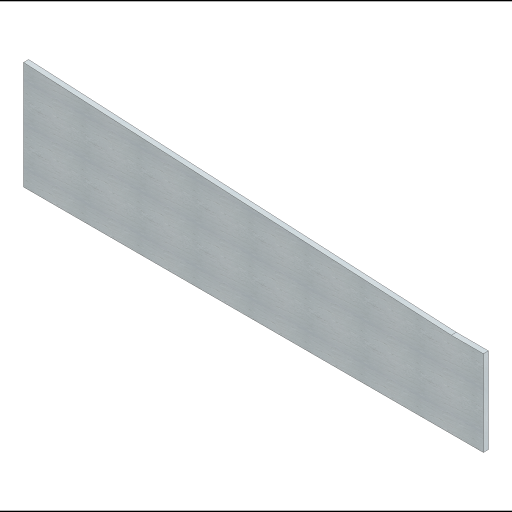
# Autodesk Inventor part: Outlet Support Leg Proto 1
Saved by Autodesk Inventor 2023 (Build 270158000, 158)
## iProperties
Created: 2023-01-19
Part Number: Outlet Support Leg Proto 1
Material: Wood (Oak)
Document SubType Name: Modeling
Designer: kamer
Density: 0.76 g/cm^3
Appearance: Wood - Painted White
Author: kamer
Autodesk Inventor part; units mm, degrees
ref_plane "YZ Plane" through (0, 0, 0) normal (1, 0, 0) x (0, 1, 0)
ref_plane "XZ Plane" through (0, 0, 0) normal (0, 1, 0) x (-1, 0, 0)
ref_plane "XY Plane" through (0, 0, 0) normal (0, 0, 1) x (1, 0, 0)
sketch "Sketch1" plane through (0, 0, 0) normal (0, 0, 1) x (1, 0, 0)
  line L0 (0, 0) -> (76.2, 0)
  line L1 (76.2, 0) -> (76.2, 203.2)
  line L2 (76.2, 203.2) -> (0, 203.2)
  line L3 (0, 203.2) -> (0, 0)
  line L4 (0, 203.2) -> (-406.4, 203.2) construction
  line L5 (0, 203.2) -> (-1016, 256.4463)
  line L6 (0, 0) -> (-1016, 0)
  line L7 (-1016, 0) -> (-1016, 256.4463)
  dimension "d0" = 203.2
  dimension "d1" = 76.2
  dimension "d2" = 3
  dimension "d3" = 1016
  constraints: 16 end point, 3 horizontal, 2 parallel, 2 perpendicular
  measures "d0" distance of L0.end L1.end
  measures "d1" distance of L1.end L2.end
  measures "d2" angle of L5 L4
  measures "d3" distance from line of L3 L5.end
extrude "Extrusion1" add sketch "Sketch1" along normal blind 11.938
body "Solid1"
